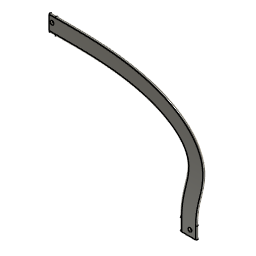
structuralThing v28 (Autodesk Fusion 360 design; units mm, degrees)
Autodesk Fusion 360 part; units mm, degrees
sketch "Sketch1" plane through (0, 0, 0) normal (1, 0, 0) x (0, 1, 0)
  spline S0 degree 5 poles (0, 0) (0.1058, 0) (0.3174, 0.0986) (0.6269, 0.542) (0.9922, 1.6752) (1.3536, 3.7189) (1.6179, 6.0396) (1.7849, 8.3197) (1.8407, 10.3115) (1.7144, 12.0439) (1.3513, 13.4682) (0.7607, 14.426) (0, 14.7714) (-0.7607, 14.426) (-1.3513, 13.4682) (-1.7144, 12.0439) (-1.8407, 10.3115) (-1.7849, 8.3197) (-1.6179, 6.0396) (-1.3536, 3.7189) (-0.9922, 1.6752) (-0.6269, 0.542) (-0.3174, 0.0986) (-0.1058, 0) (0, 0) knots 0 0 0 0 0 0 0.05 0.1 0.15 0.2 0.25 0.3 0.35 0.4 0.45 0.5 0.55 0.6 0.65 0.7 0.75 0.8 0.85 0.9 0.95 1 1 1 1 1 1
  line L0 (1.8, 7.805) -> (1.8, 11.795)
  line L1 (-1.8, 11.795) -> (-1.8, 7.805)
  line L2 (0.74, 14.6) -> (-0.74, 14.6)
  line L3 (-0.345, 0) -> (0.345, 0)
  line L4 (0.8, 10.6) -> (0.8, 8.1)
  arc A0 (0.8, 8.1) -> (2.2, 8.1) centre (1.5, 8.1) ccw
  line L5 (2.2, 8.1) -> (2.2, 10.6)
  arc A1 (2.2, 10.6) -> (0.8, 10.6) centre (1.5, 10.6) ccw
  line L6 (1.5, 10.6) -> (1.5, 8.1) construction
  line L7 (-5.6108, 0) -> (-1, 0)
  line L8 (-1, 0) -> (-1, 14.6)
  line L9 (-1, 14.6) -> (-5.6108, 14.6)
  line L10 (-5.6108, 14.6) -> (-5.6108, 0)
  point P0 (1.8, 9.8)
  point P1 (0, 14.6)
  point P2 (-1.8, 9.8)
  dimension "d1" = 9.8
  dimension "d2" = 4.8
  dimension "d3" = 3.6
  dimension "d4" = 1.8
  dimension "d7" = 3.99
  dimension "d8" = 1.48
  dimension "d9" = 0.69
  dimension "d22" = 2.5
  dimension "d23" = 0.7
  dimension "d32" = 1.5
  dimension "d33" = 4
  dimension "d50" = 1
  constraint coincident S0.start S0.end
  constraint horizontal P0 P2
  constraint vertical S0.start P1
  constraint midpoint P0 L0
  constraint vertical L0
  constraint midpoint P2 L1
  constraint vertical L1
  constraint equal L0 L1
  constraint midpoint P1 L2
  constraint midpoint S0.start L3
  constraint horizontal L2
  constraint horizontal L3
  constraint tangent L4 A0
  constraint tangent A0 L5
  constraint parallel L4 L5
  constraint tangent L5 A1
  constraint tangent L4 A1
  constraint parallel L0 L6
  constraint horizontal L7
  constraint vertical L8
  constraint horizontal L9
  constraint vertical L10
  constraint horizontal S0.start L7.end
  constraint horizontal P1 L8.end
  measures "d1" distance of S0.start P2
  measures "d2" vertical distance of P1 P2
  measures "d3" distance of P0 P2
  measures "d4" horizontal distance of P0 P1
  measures "d7" distance of L0.start L0.end
  measures "d8" distance of L2.start L2.end
  measures "d9" distance of L3.start L3.end
  measures "d22" distance of A1.centre A0.centre
  measures "d23" radius of A1
  measures "d32" horizontal distance of P1 A1.centre
  measures "d33" vertical distance of P1 A1.centre
  measures "d50" distance of S0.start L7.end
sketch "Sketch2" plane through (0, 0, 0) normal (0, 1, 0) x (1, 0, 0)
  spline S0 degree 5 poles (0, 0) (2.3895, 0) (7.6554, -0.0112) (17.0138, -0.0623) (32.1264, 0.0249) (53.6486, 1.493) (75.4441, 5.5778) (94.6141, 12.9773) (108.4792, 23.7731) (113.5969, 35.5521) (111.6509, 47.8729) (108.0834, 59.0827) (106.3787, 68.8945) (106, 76.175) (106, 80) knots 0 0 0 0 0 0 0.1 0.2 0.3 0.4 0.5 0.6 0.7 0.8 0.9 1 1 1 1 1 1
  line L0 (106, 48.0702) -> (106, 111.9298)
  line L1 (-14.7723, 0) -> (14.7723, 0)
  line L2 (88.2721, 7.1271) -> (118.1197, 34.4401)
  point P0 (103.1959, 20.7836)
  dimension "d10" = 80
  dimension "d11" = 106
  constraint coincident S0.start origin
  constraint midpoint S0.end L0
  constraint vertical L0
  constraint midpoint S0.start L1
  constraint horizontal L1
  constraint midpoint P0 L2
  measures "d10" distance of S0.end S0.start
  measures "d11" distance of S0.start S0.end
sweep "Sweep1" add profiles "Sketch1" path "Sketch2" along S0 section 1 contours S0 L4 A0 A1 L8
extrude "Extrude2" add 1 faces at (0, -0.4, 7.9981) along direction (-1, 0, 0) blind 5
extrude "Extrude3" add 1 faces at (113.9981, -0.4, -80) along direction (0, 0, -1) blind 10
sketch "Sketch3" plane through (0, 0, 0) normal (0, 1, 0) x (1, 0, 0)
  circle A0 centre (-2.5, -9) radius 1.6
  circle A1 centre (115, 85) radius 1.6
  line L0 (106, 90) -> (113.4315, 90)
  line L1 (117.257, 90) -> (120.6, 90)
  dimension "d24" = 3.2
  dimension "d25" = 3.2
  dimension "d26" = 9
  dimension "d27" = 2.5
  dimension "d51" = 5
  dimension "d53" = 9
  measures "d24" diameter of A0
  measures "d25" diameter of A1
  measures "d26" vertical distance of origin A0.centre
  measures "d27" horizontal distance of origin A0.centre
  measures "d51" vertical distance of A1.centre L1.end
  measures "d53" horizontal distance of A1.centre L0.start
extrude "Extrude4" cut sketch "Sketch3" along normal mid plane 20
equation "d22 = 4 mm - 1.5 mm"
equation "d23 = ( 1.4 / 2 ) * 1 mm"
